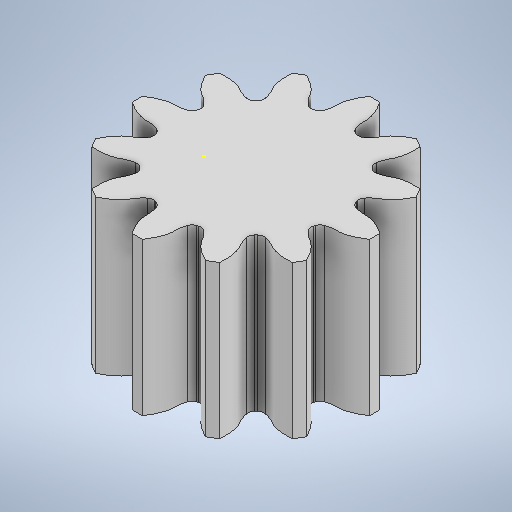
# Autodesk Inventor part: gear_3
Saved by Autodesk Inventor 2025.2 (Build 292293000, 293)
## iProperties
Created: 2025-03-25
Part Number: gear_3
Material: Generic
Document SubType Name: Modeling
Designer: Admin
Density: 1 g/cm^3
Appearance: Default
Author: Admin
Autodesk Inventor part; units mm, degrees
ref_plane "YZ Plane" through (0, 0, 0) normal (1, 0, 0) x (0, 1, 0)
ref_plane "XZ Plane" through (0, 0, 0) normal (0, 1, 0) x (-1, 0, 0)
ref_plane "XY Plane" through (0, 0, 0) normal (0, 0, 1) x (1, 0, 0)
sketch "Sketch1" plane through (0, 0, 0) normal (0, 1, 0) x (-1, 0, 0)
  arc A0 (-1.7921, 6.0379) -> (-2.4128, 6.0379) centre (-2.1025, -0.9552) ccw
  spline S0 degree 3 poles (-2.4128, 6.0379) (-2.4411, 5.9956) (-2.4962, 5.91) (-2.5737, 5.7785) (-2.6458, 5.6439) (-2.7118, 5.5063) (-2.7718, 5.3659) (-2.8243, 5.2225) (-2.8678, 5.0761) (-2.9004, 4.927) (-2.9252, 4.7759) (-2.9216, 4.6231) (-2.9181, 4.4703) (-2.9428, 4.3192) (-2.9755, 4.1702) (-3.0084, 4.0593) (-3.0293, 3.9981) (-3.0338, 3.9851) knots 0.009806 0.009806 0.009806 0.009806 0.07852 0.147233 0.215945 0.284657 0.353368 0.422077 0.490783 0.559487 0.628183 0.696834 0.765485 0.834181 0.902886 0.971592 0.990196 0.990196 0.990196 0.990196
  arc A1 (-3.3051, 3.7361) -> (-3.0338, 3.9851) centre (-3.402, 4.1139) ccw
  arc A2 (-3.3051, 3.7361) -> (-3.4066, 3.7089) centre (-2.1025, -0.9552) ccw
  arc A3 (-3.7661, 3.7889) -> (-3.4066, 3.7089) centre (-3.5116, 4.0845) ccw
  spline S1 degree 3 poles (-3.7661, 3.7889) (-3.7765, 3.7979) (-3.8252, 3.8405) (-3.9091, 3.92) (-4.0119, 4.0327) (-4.1089, 4.1512) (-4.1822, 4.2853) (-4.2556, 4.4194) (-4.3526, 4.5379) (-4.4554, 4.6507) (-4.5663, 4.7557) (-4.6834, 4.8536) (-4.8056, 4.9452) (-4.9315, 5.0315) (-5.0612, 5.112) (-5.1941, 5.1871) (-5.2846, 5.2337) (-5.3303, 5.2562) knots 0.009805 0.009805 0.009805 0.009805 0.028409 0.097115 0.165819 0.234515 0.303166 0.371817 0.440513 0.509218 0.577924 0.646632 0.715343 0.784055 0.852768 0.921481 0.990194 0.990194 0.990194 0.990194
  arc A4 (-5.3303, 5.2562) -> (-5.8678, 4.9458) centre (-2.1025, -0.9552) ccw
  spline S2 degree 3 poles (-5.8678, 4.9458) (-5.8712, 4.8951) (-5.8761, 4.7934) (-5.8775, 4.6408) (-5.8726, 4.4882) (-5.8609, 4.3359) (-5.8426, 4.1844) (-5.8164, 4.034) (-5.7809, 3.8854) (-5.7347, 3.74) (-5.6805, 3.5967) (-5.6011, 3.4662) (-5.5216, 3.3356) (-5.4675, 3.1924) (-5.4212, 3.047) (-5.3943, 2.9345) (-5.3818, 2.8711) (-5.3792, 2.8576) knots 0.009806 0.009806 0.009806 0.009806 0.07852 0.147233 0.215945 0.284657 0.353368 0.422077 0.490783 0.559487 0.628183 0.696834 0.765485 0.834181 0.902886 0.971592 0.990196 0.990196 0.990196 0.990196
  arc A5 (-5.4897, 2.5062) -> (-5.3792, 2.8576) centre (-5.7624, 2.785) ccw
  arc A6 (-5.4897, 2.5062) -> (-5.5639, 2.432) centre (-2.1025, -0.9552) ccw
  arc A7 (-5.9153, 2.3215) -> (-5.5639, 2.432) centre (-5.8427, 2.7047) ccw
  spline S3 degree 3 poles (-5.9153, 2.3215) (-5.9288, 2.3241) (-5.9922, 2.3366) (-6.1047, 2.3635) (-6.2501, 2.4098) (-6.3933, 2.4639) (-6.5239, 2.5434) (-6.6544, 2.6228) (-6.7977, 2.677) (-6.9431, 2.7232) (-7.0917, 2.7587) (-7.2421, 2.7849) (-7.3936, 2.8032) (-7.5459, 2.8149) (-7.6985, 2.8198) (-7.8511, 2.8184) (-7.9528, 2.8135) (-8.0035, 2.8101) knots 0.009805 0.009805 0.009805 0.009805 0.028409 0.097115 0.165819 0.234515 0.303166 0.371817 0.440513 0.509218 0.577924 0.646632 0.715343 0.784055 0.852768 0.921481 0.990194 0.990194 0.990194 0.990194
  arc A8 (-8.0035, 2.8101) -> (-8.3139, 2.2726) centre (-2.1025, -0.9552) ccw
  spline S4 degree 3 poles (-8.3139, 2.2726) (-8.2914, 2.2269) (-8.2448, 2.1364) (-8.1697, 2.0035) (-8.0892, 1.8738) (-8.0029, 1.7479) (-7.9113, 1.6257) (-7.8134, 1.5086) (-7.7084, 1.3977) (-7.5956, 1.2949) (-7.4771, 1.1979) (-7.343, 1.1245) (-7.2089, 1.0512) (-7.0904, 0.9542) (-6.9777, 0.8514) (-6.8982, 0.7675) (-6.8556, 0.7188) (-6.8466, 0.7084) knots 0.009806 0.009806 0.009806 0.009806 0.07852 0.147233 0.215945 0.284657 0.353368 0.422077 0.490783 0.559487 0.628183 0.696834 0.765485 0.834181 0.902886 0.971592 0.990196 0.990196 0.990196 0.990196
  arc A9 (-6.7666, 0.3489) -> (-6.8466, 0.7084) centre (-7.1422, 0.4539) ccw
  arc A10 (-6.7666, 0.3489) -> (-6.7938, 0.2474) centre (-2.1025, -0.9552) ccw
  arc A11 (-7.0428, -0.0239) -> (-6.7938, 0.2474) centre (-7.1716, 0.3443) ccw
  spline S5 degree 3 poles (-7.0428, -0.0239) (-7.0558, -0.0284) (-7.117, -0.0493) (-7.2279, -0.0822) (-7.3769, -0.1149) (-7.528, -0.1396) (-7.6808, -0.1361) (-7.8336, -0.1325) (-7.9847, -0.1573) (-8.1338, -0.1899) (-8.2802, -0.2334) (-8.4236, -0.2859) (-8.564, -0.3459) (-8.7016, -0.4119) (-8.8362, -0.484) (-8.9677, -0.5615) (-9.0533, -0.6166) (-9.0956, -0.6449) knots 0.009805 0.009805 0.009805 0.009805 0.028409 0.097115 0.165819 0.234515 0.303166 0.371817 0.440513 0.509218 0.577924 0.646632 0.715343 0.784055 0.852768 0.921481 0.990194 0.990194 0.990194 0.990194
  arc A12 (-9.0956, -0.6449) -> (-9.0956, -1.2656) centre (-2.1025, -0.9552) ccw
  spline S6 degree 3 poles (-9.0956, -1.2656) (-9.0533, -1.2939) (-8.9677, -1.3489) (-8.8362, -1.4265) (-8.7016, -1.4985) (-8.564, -1.5645) (-8.4236, -1.6245) (-8.2802, -1.677) (-8.1338, -1.7205) (-7.9847, -1.7532) (-7.8336, -1.7779) (-7.6808, -1.7744) (-7.528, -1.7708) (-7.3769, -1.7956) (-7.2279, -1.8282) (-7.117, -1.8612) (-7.0558, -1.882) (-7.0428, -1.8866) knots 0.009806 0.009806 0.009806 0.009806 0.07852 0.147233 0.215945 0.284657 0.353368 0.422077 0.490783 0.559487 0.628183 0.696834 0.765485 0.834181 0.902886 0.971592 0.990196 0.990196 0.990196 0.990196
  arc A13 (-6.7938, -2.1579) -> (-7.0428, -1.8866) centre (-7.1716, -2.2547) ccw
  arc A14 (-6.7938, -2.1579) -> (-6.7666, -2.2593) centre (-2.1025, -0.9552) ccw
  arc A15 (-6.8466, -2.6188) -> (-6.7666, -2.2593) centre (-7.1422, -2.3644) ccw
  spline S7 degree 3 poles (-6.8466, -2.6188) (-6.8556, -2.6292) (-6.8982, -2.6779) (-6.9777, -2.7618) (-7.0904, -2.8646) (-7.2089, -2.9616) (-7.343, -3.035) (-7.4771, -3.1083) (-7.5956, -3.2053) (-7.7084, -3.3081) (-7.8134, -3.419) (-7.9113, -3.5362) (-8.0029, -3.6583) (-8.0892, -3.7843) (-8.1697, -3.914) (-8.2448, -4.0469) (-8.2914, -4.1374) (-8.3139, -4.183) knots 0.009805 0.009805 0.009805 0.009805 0.028409 0.097115 0.165819 0.234515 0.303166 0.371817 0.440513 0.509218 0.577924 0.646632 0.715343 0.784055 0.852768 0.921481 0.990194 0.990194 0.990194 0.990194
  arc A16 (-8.3139, -4.183) -> (-8.0035, -4.7205) centre (-2.1025, -0.9552) ccw
  spline S8 degree 3 poles (-8.0035, -4.7205) (-7.9528, -4.7239) (-7.8511, -4.7288) (-7.6985, -4.7302) (-7.5459, -4.7253) (-7.3936, -4.7136) (-7.2421, -4.6954) (-7.0917, -4.6692) (-6.9431, -4.6336) (-6.7977, -4.5874) (-6.6544, -4.5333) (-6.5239, -4.4538) (-6.3933, -4.3743) (-6.2501, -4.3202) (-6.1047, -4.274) (-5.9922, -4.2471) (-5.9288, -4.2345) (-5.9153, -4.232) knots 0.009806 0.009806 0.009806 0.009806 0.07852 0.147233 0.215945 0.284657 0.353368 0.422077 0.490783 0.559487 0.628183 0.696834 0.765485 0.834181 0.902886 0.971592 0.990196 0.990196 0.990196 0.990196
  arc A17 (-5.5639, -4.3424) -> (-5.9153, -4.232) centre (-5.8427, -4.6152) ccw
  arc A18 (-5.5639, -4.3424) -> (-5.4897, -4.4167) centre (-2.1025, -0.9552) ccw
  arc A19 (-5.3792, -4.768) -> (-5.4897, -4.4167) centre (-5.7624, -4.6954) ccw
  spline S9 degree 3 poles (-5.3792, -4.768) (-5.3818, -4.7815) (-5.3943, -4.845) (-5.4212, -4.9574) (-5.4675, -5.1028) (-5.5216, -5.2461) (-5.6011, -5.3766) (-5.6805, -5.5072) (-5.7347, -5.6504) (-5.7809, -5.7958) (-5.8164, -5.9444) (-5.8426, -6.0948) (-5.8609, -6.2464) (-5.8726, -6.3986) (-5.8775, -6.5512) (-5.8761, -6.7038) (-5.8712, -6.8055) (-5.8678, -6.8563) knots 0.009805 0.009805 0.009805 0.009805 0.028409 0.097115 0.165819 0.234515 0.303166 0.371817 0.440513 0.509218 0.577924 0.646632 0.715343 0.784055 0.852768 0.921481 0.990194 0.990194 0.990194 0.990194
  arc A20 (-5.8678, -6.8563) -> (-5.3303, -7.1666) centre (-2.1025, -0.9552) ccw
  spline S10 degree 3 poles (-5.3303, -7.1666) (-5.2846, -7.1441) (-5.1941, -7.0975) (-5.0612, -7.0224) (-4.9315, -6.9419) (-4.8056, -6.8557) (-4.6834, -6.7641) (-4.5663, -6.6662) (-4.4554, -6.5611) (-4.3526, -6.4484) (-4.2556, -6.3299) (-4.1822, -6.1958) (-4.1089, -6.0617) (-4.0119, -5.9432) (-3.9091, -5.8304) (-3.8252, -5.7509) (-3.7765, -5.7083) (-3.7661, -5.6994) knots 0.009806 0.009806 0.009806 0.009806 0.07852 0.147233 0.215945 0.284657 0.353368 0.422077 0.490783 0.559487 0.628183 0.696834 0.765485 0.834181 0.902886 0.971592 0.990196 0.990196 0.990196 0.990196
  arc A21 (-3.4066, -5.6193) -> (-3.7661, -5.6994) centre (-3.5116, -5.9949) ccw
  arc A22 (-3.4066, -5.6193) -> (-3.3051, -5.6465) centre (-2.1025, -0.9552) ccw
  arc A23 (-3.0338, -5.8956) -> (-3.3051, -5.6465) centre (-3.402, -6.0243) ccw
  spline S11 degree 3 poles (-3.0338, -5.8956) (-3.0293, -5.9086) (-3.0084, -5.9698) (-2.9755, -6.0806) (-2.9428, -6.2296) (-2.9181, -6.3808) (-2.9216, -6.5335) (-2.9252, -6.6863) (-2.9004, -6.8375) (-2.8678, -6.9865) (-2.8243, -7.1329) (-2.7718, -7.2763) (-2.7118, -7.4167) (-2.6458, -7.5544) (-2.5737, -7.689) (-2.4962, -7.8205) (-2.4411, -7.9061) (-2.4128, -7.9483) knots 0.009805 0.009805 0.009805 0.009805 0.028409 0.097115 0.165819 0.234515 0.303166 0.371817 0.440513 0.509218 0.577924 0.646632 0.715343 0.784055 0.852768 0.921481 0.990194 0.990194 0.990194 0.990194
  arc A24 (-2.4128, -7.9483) -> (-1.7921, -7.9483) centre (-2.1025, -0.9552) ccw
  spline S12 degree 3 poles (-1.7921, -7.9483) (-1.7638, -7.9061) (-1.7088, -7.8205) (-1.6312, -7.689) (-1.5592, -7.5544) (-1.4932, -7.4167) (-1.4332, -7.2763) (-1.3807, -7.1329) (-1.3372, -6.9865) (-1.3045, -6.8375) (-1.2798, -6.6863) (-1.2833, -6.5335) (-1.2869, -6.3808) (-1.2621, -6.2296) (-1.2295, -6.0806) (-1.1965, -5.9698) (-1.1757, -5.9086) (-1.1711, -5.8956) knots 0.009806 0.009806 0.009806 0.009806 0.07852 0.147233 0.215945 0.284657 0.353368 0.422077 0.490783 0.559487 0.628183 0.696834 0.765485 0.834181 0.902886 0.971592 0.990196 0.990196 0.990196 0.990196
  arc A25 (-0.8998, -5.6465) -> (-1.1711, -5.8956) centre (-0.803, -6.0243) ccw
  arc A26 (-0.8998, -5.6465) -> (-0.7984, -5.6193) centre (-2.1025, -0.9552) ccw
  arc A27 (-0.4389, -5.6994) -> (-0.7984, -5.6193) centre (-0.6933, -5.9949) ccw
  spline S13 degree 3 poles (-0.4389, -5.6994) (-0.4285, -5.7083) (-0.3798, -5.7509) (-0.2959, -5.8304) (-0.1931, -5.9432) (-0.0961, -6.0617) (-0.0227, -6.1958) (0.0506, -6.3299) (0.1476, -6.4484) (0.2504, -6.5611) (0.3613, -6.6662) (0.4785, -6.7641) (0.6006, -6.8557) (0.7266, -6.9419) (0.8563, -7.0224) (0.9892, -7.0975) (1.0797, -7.1441) (1.1253, -7.1666) knots 0.009805 0.009805 0.009805 0.009805 0.028409 0.097115 0.165819 0.234515 0.303166 0.371817 0.440513 0.509218 0.577924 0.646632 0.715343 0.784055 0.852768 0.921481 0.990194 0.990194 0.990194 0.990194
  arc A28 (1.1253, -7.1666) -> (1.6628, -6.8563) centre (-2.1025, -0.9552) ccw
  spline S14 degree 3 poles (1.6628, -6.8563) (1.6662, -6.8055) (1.6711, -6.7038) (1.6725, -6.5512) (1.6676, -6.3986) (1.6559, -6.2464) (1.6377, -6.0948) (1.6115, -5.9444) (1.5759, -5.7958) (1.5297, -5.6504) (1.4756, -5.5072) (1.3961, -5.3766) (1.3166, -5.2461) (1.2625, -5.1028) (1.2163, -4.9574) (1.1894, -4.845) (1.1768, -4.7815) (1.1743, -4.768) knots 0.009806 0.009806 0.009806 0.009806 0.07852 0.147233 0.215945 0.284657 0.353368 0.422077 0.490783 0.559487 0.628183 0.696834 0.765485 0.834181 0.902886 0.971592 0.990196 0.990196 0.990196 0.990196
  arc A29 (1.2847, -4.4167) -> (1.1743, -4.768) centre (1.5575, -4.6954) ccw
  arc A30 (1.2847, -4.4167) -> (1.359, -4.3424) centre (-2.1025, -0.9552) ccw
  arc A31 (1.7103, -4.232) -> (1.359, -4.3424) centre (1.6377, -4.6152) ccw
  spline S15 degree 3 poles (1.7103, -4.232) (1.7238, -4.2345) (1.7873, -4.2471) (1.8997, -4.274) (2.0451, -4.3202) (2.1884, -4.3743) (2.3189, -4.4538) (2.4495, -4.5333) (2.5927, -4.5874) (2.7381, -4.6336) (2.8867, -4.6692) (3.0371, -4.6954) (3.1887, -4.7136) (3.3409, -4.7253) (3.4935, -4.7302) (3.6461, -4.7288) (3.7478, -4.7239) (3.7986, -4.7205) knots 0.009805 0.009805 0.009805 0.009805 0.028409 0.097115 0.165819 0.234515 0.303166 0.371817 0.440513 0.509218 0.577924 0.646632 0.715343 0.784055 0.852768 0.921481 0.990194 0.990194 0.990194 0.990194
  arc A32 (3.7986, -4.7205) -> (4.1089, -4.183) centre (-2.1025, -0.9552) ccw
  spline S16 degree 3 poles (4.1089, -4.183) (4.0864, -4.1374) (4.0398, -4.0469) (3.9647, -3.914) (3.8842, -3.7843) (3.798, -3.6583) (3.7064, -3.5362) (3.6085, -3.419) (3.5034, -3.3081) (3.3907, -3.2053) (3.2722, -3.1083) (3.1381, -3.035) (3.004, -2.9616) (2.8855, -2.8646) (2.7727, -2.7618) (2.6932, -2.6779) (2.6506, -2.6292) (2.6416, -2.6188) knots 0.009806 0.009806 0.009806 0.009806 0.07852 0.147233 0.215945 0.284657 0.353368 0.422077 0.490783 0.559487 0.628183 0.696834 0.765485 0.834181 0.902886 0.971592 0.990196 0.990196 0.990196 0.990196
  arc A33 (2.5616, -2.2593) -> (2.6416, -2.6188) centre (2.9372, -2.3644) ccw
  arc A34 (2.5616, -2.2593) -> (2.5888, -2.1579) centre (-2.1025, -0.9552) ccw
  arc A35 (2.8378, -1.8866) -> (2.5888, -2.1579) centre (2.9666, -2.2547) ccw
  spline S17 degree 3 poles (2.8378, -1.8866) (2.8509, -1.882) (2.9121, -1.8612) (3.0229, -1.8282) (3.1719, -1.7956) (3.3231, -1.7708) (3.4758, -1.7744) (3.6286, -1.7779) (3.7798, -1.7532) (3.9288, -1.7205) (4.0752, -1.677) (4.2186, -1.6245) (4.359, -1.5645) (4.4967, -1.4985) (4.6313, -1.4265) (4.7628, -1.3489) (4.8484, -1.2939) (4.8906, -1.2656) knots 0.009805 0.009805 0.009805 0.009805 0.028409 0.097115 0.165819 0.234515 0.303166 0.371817 0.440513 0.509218 0.577924 0.646632 0.715343 0.784055 0.852768 0.921481 0.990194 0.990194 0.990194 0.990194
  arc A36 (4.8906, -1.2656) -> (4.8906, -0.6449) centre (-2.1025, -0.9552) ccw
  spline S18 degree 3 poles (4.8906, -0.6449) (4.8484, -0.6166) (4.7628, -0.5615) (4.6313, -0.484) (4.4967, -0.4119) (4.359, -0.3459) (4.2186, -0.2859) (4.0752, -0.2334) (3.9288, -0.1899) (3.7798, -0.1573) (3.6286, -0.1325) (3.4758, -0.1361) (3.3231, -0.1396) (3.1719, -0.1149) (3.0229, -0.0822) (2.9121, -0.0493) (2.8509, -0.0284) (2.8378, -0.0239) knots 0.009806 0.009806 0.009806 0.009806 0.07852 0.147233 0.215945 0.284657 0.353368 0.422077 0.490783 0.559487 0.628183 0.696834 0.765485 0.834181 0.902886 0.971592 0.990196 0.990196 0.990196 0.990196
  arc A37 (2.5888, 0.2474) -> (2.8378, -0.0239) centre (2.9666, 0.3443) ccw
  arc A38 (2.5888, 0.2474) -> (2.5616, 0.3489) centre (-2.1025, -0.9552) ccw
  arc A39 (2.6416, 0.7084) -> (2.5616, 0.3489) centre (2.9372, 0.4539) ccw
  spline S19 degree 3 poles (2.6416, 0.7084) (2.6506, 0.7188) (2.6932, 0.7675) (2.7727, 0.8514) (2.8855, 0.9542) (3.004, 1.0512) (3.1381, 1.1245) (3.2722, 1.1979) (3.3907, 1.2949) (3.5034, 1.3977) (3.6085, 1.5086) (3.7064, 1.6257) (3.798, 1.7479) (3.8842, 1.8738) (3.9647, 2.0035) (4.0398, 2.1364) (4.0864, 2.2269) (4.1089, 2.2726) knots 0.009805 0.009805 0.009805 0.009805 0.028409 0.097115 0.165819 0.234515 0.303166 0.371817 0.440513 0.509218 0.577924 0.646632 0.715343 0.784055 0.852768 0.921481 0.990194 0.990194 0.990194 0.990194
  arc A40 (4.1089, 2.2726) -> (3.7986, 2.8101) centre (-2.1025, -0.9552) ccw
  spline S20 degree 3 poles (3.7986, 2.8101) (3.7478, 2.8135) (3.6461, 2.8184) (3.4935, 2.8198) (3.3409, 2.8149) (3.1887, 2.8032) (3.0371, 2.7849) (2.8867, 2.7587) (2.7381, 2.7232) (2.5927, 2.677) (2.4495, 2.6228) (2.3189, 2.5434) (2.1884, 2.4639) (2.0451, 2.4098) (1.8997, 2.3635) (1.7873, 2.3366) (1.7238, 2.3241) (1.7103, 2.3215) knots 0.009806 0.009806 0.009806 0.009806 0.07852 0.147233 0.215945 0.284657 0.353368 0.422077 0.490783 0.559487 0.628183 0.696834 0.765485 0.834181 0.902886 0.971592 0.990196 0.990196 0.990196 0.990196
  arc A41 (1.359, 2.432) -> (1.7103, 2.3215) centre (1.6377, 2.7047) ccw
  arc A42 (1.359, 2.432) -> (1.2847, 2.5062) centre (-2.1025, -0.9552) ccw
  arc A43 (1.1743, 2.8576) -> (1.2847, 2.5062) centre (1.5575, 2.785) ccw
  spline S21 degree 3 poles (1.1743, 2.8576) (1.1768, 2.8711) (1.1894, 2.9345) (1.2163, 3.047) (1.2625, 3.1924) (1.3166, 3.3356) (1.3961, 3.4662) (1.4756, 3.5967) (1.5297, 3.74) (1.5759, 3.8854) (1.6115, 4.034) (1.6377, 4.1844) (1.6559, 4.3359) (1.6676, 4.4882) (1.6725, 4.6408) (1.6711, 4.7934) (1.6662, 4.8951) (1.6628, 4.9458) knots 0.009805 0.009805 0.009805 0.009805 0.028409 0.097115 0.165819 0.234515 0.303166 0.371817 0.440513 0.509218 0.577924 0.646632 0.715343 0.784055 0.852768 0.921481 0.990194 0.990194 0.990194 0.990194
  arc A44 (1.6628, 4.9458) -> (1.1253, 5.2562) centre (-2.1025, -0.9552) ccw
  spline S22 degree 3 poles (1.1253, 5.2562) (1.0797, 5.2337) (0.9892, 5.1871) (0.8563, 5.112) (0.7266, 5.0315) (0.6006, 4.9452) (0.4785, 4.8536) (0.3613, 4.7557) (0.2504, 4.6507) (0.1476, 4.5379) (0.0506, 4.4194) (-0.0227, 4.2853) (-0.0961, 4.1512) (-0.1931, 4.0327) (-0.2959, 3.92) (-0.3798, 3.8405) (-0.4285, 3.7979) (-0.4389, 3.7889) knots 0.009806 0.009806 0.009806 0.009806 0.07852 0.147233 0.215945 0.284657 0.353368 0.422077 0.490783 0.559487 0.628183 0.696834 0.765485 0.834181 0.902886 0.971592 0.990196 0.990196 0.990196 0.990196
  arc A45 (-0.7984, 3.7089) -> (-0.4389, 3.7889) centre (-0.6933, 4.0845) ccw
  arc A46 (-0.7984, 3.7089) -> (-0.8998, 3.7361) centre (-2.1025, -0.9552) ccw
  arc A47 (-1.1711, 3.9851) -> (-0.8998, 3.7361) centre (-0.803, 4.1139) ccw
  spline S23 degree 3 poles (-1.1711, 3.9851) (-1.1757, 3.9981) (-1.1965, 4.0593) (-1.2295, 4.1702) (-1.2621, 4.3192) (-1.2869, 4.4703) (-1.2833, 4.6231) (-1.2798, 4.7759) (-1.3045, 4.927) (-1.3372, 5.0761) (-1.3807, 5.2225) (-1.4332, 5.3659) (-1.4932, 5.5063) (-1.5592, 5.6439) (-1.6312, 5.7785) (-1.7088, 5.91) (-1.7638, 5.9956) (-1.7921, 6.0379) knots 0.009805 0.009805 0.009805 0.009805 0.028409 0.097115 0.165819 0.234515 0.303166 0.371817 0.440513 0.509218 0.577924 0.646632 0.715343 0.784055 0.852768 0.921481 0.990194 0.990194 0.990194 0.990194
  circle A48 centre (-2.1025, -0.9552) radius 2.5
  point P0 (0, 0)
  dimension "d2" = 5
  constraints: 96 point on circle, 49 centre point, 1 coincident, 48 other
  measures "d2" diameter of A48
extrude "Extrusion1" add sketch "Sketch1" along normal blind 9 contours S23 A47 A46 A45 S22 A44 S21 A43 A42 A41 S20 A40 S19 A39 A38 A37 S18 A36 S17 A35 A34 A33 S16 A32 S15 A31 A30 A29 S14 A28 S13 A27 A26 A25 S12 A24 S11 A23 A22 A21 S10 A20 S9 A19 A18 A17 S8 A16 S7 A15 A14 A13 S6 A12 S5 A11 A10 A9 S4 A8 S3 A7 A6 A5 S2 A4 S1 A3 A2 A1 S0 A0 | A48
sketch "Sketch2" plane through (0, 9, 0) normal (0, 1, 0) x (1, 0, 0)
  point P0 (0, 0)
body "Solid1"
